Autodesk Inventor part; units mm, degrees
(part 2 of 3)
  spline S117 degree 2 poles (10.1065, 124.379) (9.1972, 124.379) (8.3459, 125.7919) (8.3459, 127.2404) knots 0 0 0 1 2 2 2
  spline S118 degree 2 poles (8.3459, 127.2404) (8.3459, 128.7291) (9.2061, 130.1063) (10.1065, 130.1063) knots 0 0 0 1 2 2 2
  spline S119 degree 2 poles (10.1065, 130.1063) (11.0112, 130.1063) (11.8625, 128.68) (11.8625, 127.2449) knots 0 0 0 1 2 2 2
  spline S120 degree 2 poles (10.9176, 125.569) (11.0246, 125.8409) (11.1138, 126.6788) (11.1138, 127.2449) knots 0 0 0 1 2 2 2
  spline S121 degree 2 poles (11.1138, 127.2449) (11.1138, 127.8109) (11.0246, 128.6444) (10.9132, 128.9252) knots 0 0 0 1 2 2 2
  spline S122 degree 2 poles (10.9132, 128.9252) (10.8018, 129.206) (10.414, 129.4957) (10.1065, 129.4957) knots 0 0 0 1 2 2 2
  spline S123 degree 2 poles (10.1065, 129.4957) (9.7989, 129.4957) (9.4022, 129.206) (9.2864, 128.9163) knots 0 0 0 1 2 2 2
  spline S124 degree 2 poles (9.2864, 128.9163) (9.1749, 128.6355) (9.0947, 127.7797) (9.0947, 127.2404) knots 0 0 0 1 2 2 2
  spline S125 degree 2 poles (9.0947, 127.2404) (9.0947, 126.661) (9.166, 125.8855) (9.2819, 125.5824) knots 0 0 0 1 2 2 2
  spline S126 degree 2 poles (9.2819, 125.5824) (9.3889, 125.2971) (9.7856, 124.9896) (10.1065, 124.9896) knots 0 0 0 1 2 2 2
  spline S127 degree 2 poles (10.1065, 124.9896) (10.4095, 124.9896) (10.8062, 125.2793) (10.9176, 125.569) knots 0 0 0 1 2 2 2
  line L151 (3.304, 115.002) -> (0.6208, 115.002)
  line L152 (0.6208, 115.002) -> (0.6208, 115.5635)
  line L153 (0.6208, 115.5635) -> (1.6192, 115.5635)
  line L154 (1.6192, 115.5635) -> (1.6192, 119.2495)
  line L155 (1.6192, 119.2495) -> (0.6208, 119.2495)
  line L156 (0.6208, 119.2495) -> (0.6208, 119.7532)
  spline S128 degree 2 poles (0.6208, 119.7532) (1.1869, 119.7532) (1.7217, 120.0741) (1.7574, 120.5198) knots 0 0 0 1 2 2 2
  line L157 (1.7574, 120.5198) -> (2.3279, 120.5198)
  line L158 (2.3279, 120.5198) -> (2.3279, 115.5635)
  line L159 (2.3279, 115.5635) -> (3.304, 115.5635)
  line L160 (3.304, 115.5635) -> (3.304, 115.002)
  spline S129 degree 2 poles (7.7387, 117.752) (7.7387, 116.2722) (6.8785, 114.8861) (5.9827, 114.8861) knots 0 0 0 1 2 2 2
  spline S130 degree 2 poles (5.9827, 114.8861) (5.0734, 114.8861) (4.2221, 116.299) (4.2221, 117.7475) knots 0 0 0 1 2 2 2
  spline S131 degree 2 poles (4.2221, 117.7475) (4.2221, 119.2362) (5.0823, 120.6134) (5.9827, 120.6134) knots 0 0 0 1 2 2 2
  spline S132 degree 2 poles (5.9827, 120.6134) (6.8874, 120.6134) (7.7387, 119.1871) (7.7387, 117.752) knots 0 0 0 1 2 2 2
  spline S133 degree 2 poles (6.7938, 116.0761) (6.9008, 116.348) (6.99, 117.1859) (6.99, 117.752) knots 0 0 0 1 2 2 2
  spline S134 degree 2 poles (6.99, 117.752) (6.99, 118.318) (6.9008, 119.1515) (6.7894, 119.4323) knots 0 0 0 1 2 2 2
  spline S135 degree 2 poles (6.7894, 119.4323) (6.678, 119.7131) (6.2902, 120.0028) (5.9827, 120.0028) knots 0 0 0 1 2 2 2
  spline S136 degree 2 poles (5.9827, 120.0028) (5.6751, 120.0028) (5.2784, 119.7131) (5.1626, 119.4233) knots 0 0 0 1 2 2 2
  spline S137 degree 2 poles (5.1626, 119.4233) (5.0511, 119.1426) (4.9709, 118.2868) (4.9709, 117.7475) knots 0 0 0 1 2 2 2
  spline S138 degree 2 poles (4.9709, 117.7475) (4.9709, 117.1681) (5.0422, 116.3926) (5.1581, 116.0895) knots 0 0 0 1 2 2 2
  spline S139 degree 2 poles (5.1581, 116.0895) (5.2651, 115.8042) (5.6617, 115.4967) (5.9827, 115.4967) knots 0 0 0 1 2 2 2
  spline S140 degree 2 poles (5.9827, 115.4967) (6.2857, 115.4967) (6.6824, 115.7864) (6.7938, 116.0761) knots 0 0 0 1 2 2 2
  spline S141 degree 2 poles (11.866, 117.752) (11.866, 116.2722) (11.0058, 114.8861) (10.1099, 114.8861) knots 0 0 0 1 2 2 2
  spline S142 degree 2 poles (10.1099, 114.8861) (9.2006, 114.8861) (8.3494, 116.299) (8.3494, 117.7475) knots 0 0 0 1 2 2 2
  spline S143 degree 2 poles (8.3494, 117.7475) (8.3494, 119.2362) (9.2096, 120.6134) (10.1099, 120.6134) knots 0 0 0 1 2 2 2
  spline S144 degree 2 poles (10.1099, 120.6134) (11.0147, 120.6134) (11.866, 119.1871) (11.866, 117.752) knots 0 0 0 1 2 2 2
  spline S145 degree 2 poles (10.9211, 116.0761) (11.028, 116.348) (11.1172, 117.1859) (11.1172, 117.752) knots 0 0 0 1 2 2 2
  spline S146 degree 2 poles (11.1172, 117.752) (11.1172, 118.318) (11.028, 119.1515) (10.9166, 119.4323) knots 0 0 0 1 2 2 2
  spline S147 degree 2 poles (10.9166, 119.4323) (10.8052, 119.7131) (10.4174, 120.0028) (10.1099, 120.0028) knots 0 0 0 1 2 2 2
  spline S148 degree 2 poles (10.1099, 120.0028) (9.8023, 120.0028) (9.4057, 119.7131) (9.2898, 119.4233) knots 0 0 0 1 2 2 2
  spline S149 degree 2 poles (9.2898, 119.4233) (9.1784, 119.1426) (9.0981, 118.2868) (9.0981, 117.7475) knots 0 0 0 1 2 2 2
  spline S150 degree 2 poles (9.0981, 117.7475) (9.0981, 117.1681) (9.1694, 116.3926) (9.2853, 116.0895) knots 0 0 0 1 2 2 2
  spline S151 degree 2 poles (9.2853, 116.0895) (9.3923, 115.8042) (9.789, 115.4967) (10.1099, 115.4967) knots 0 0 0 1 2 2 2
  spline S152 degree 2 poles (10.1099, 115.4967) (10.413, 115.4967) (10.8096, 115.7864) (10.9211, 116.0761) knots 0 0 0 1 2 2 2
  spline S153 degree 2 poles (0.4266, 108.238) (0.4266, 108.6614) (0.7029, 109.3657) (0.9436, 109.6197) knots 0 0 0 1 2 2 2
  spline S154 degree 2 poles (0.9436, 109.6197) (1.1709, 109.8648) (1.835, 110.1367) (2.1737, 110.1367) knots 0 0 0 1 2 2 2
  spline S155 degree 2 poles (2.1737, 110.1367) (2.5526, 110.1367) (3.1676, 109.8827) (3.395, 109.642) knots 0 0 0 1 2 2 2
  spline S156 degree 2 poles (3.395, 109.642) (3.6802, 109.3389) (3.9922, 108.3584) (3.9922, 107.6051) knots 0 0 0 1 2 2 2
  spline S157 degree 2 poles (3.9922, 107.6051) (3.9922, 106.9232) (3.6847, 105.702) (3.386, 105.2964) knots 0 0 0 1 2 2 2
  spline S158 degree 2 poles (3.386, 105.2964) (3.0696, 104.8685) (2.1782, 104.4183) (1.5275, 104.4183) knots 0 0 0 1 2 2 2
  spline S159 degree 2 poles (1.5275, 104.4183) (1.3804, 104.4183) (1.0461, 104.4495) (0.9035, 104.4941) knots 0 0 0 1 2 2 2
  line L161 (0.9035, 104.4941) -> (0.9035, 105.2028)
  line L162 (0.9035, 105.2028) -> (0.9391, 105.2028)
  spline S160 degree 2 poles (0.9391, 105.2028) (1.0327, 105.1493) (1.4249, 105.0557) (1.6255, 105.0557) knots 0 0 0 1 2 2 2
  spline S161 degree 2 poles (1.6255, 105.0557) (2.3475, 105.0557) (3.1721, 106.0095) (3.23, 106.892) knots 0 0 0 1 2 2 2
  spline S162 degree 2 poles (3.23, 106.892) (2.9359, 106.6914) (2.401, 106.5087) (2.0846, 106.5087) knots 0 0 0 1 2 2 2
  spline S163 degree 2 poles (2.0846, 106.5087) (1.7815, 106.5087) (1.2779, 106.6424) (1.0238, 106.8341) knots 0 0 0 1 2 2 2
  spline S164 degree 2 poles (1.0238, 106.8341) (0.7296, 107.0614) (0.4266, 107.7522) (0.4266, 108.238) knots 0 0 0 1 2 2 2
  spline S165 degree 2 poles (3.2479, 107.77) (3.2479, 108.3272) (3.0428, 109.0314) (2.8601, 109.223) knots 0 0 0 1 2 2 2
  spline S166 degree 2 poles (2.8601, 109.223) (2.6997, 109.4013) (2.3654, 109.535) (2.1693, 109.535) knots 0 0 0 1 2 2 2
  spline S167 degree 2 poles (2.1693, 109.535) (1.7146, 109.535) (1.1753, 108.8843) (1.1753, 108.2692) knots 0 0 0 1 2 2 2
  spline S168 degree 2 poles (1.1753, 108.2692) (1.1753, 107.9216) (1.3536, 107.4714) (1.5497, 107.311) knots 0 0 0 1 2 2 2
  spline S169 degree 2 poles (1.5497, 107.311) (1.6924, 107.1951) (2.0445, 107.1193) (2.2495, 107.1193) knots 0 0 0 1 2 2 2
  spline S170 degree 2 poles (2.2495, 107.1193) (2.4857, 107.1193) (3.0295, 107.2842) (3.2345, 107.4224) knots 0 0 0 1 2 2 2
  spline S171 degree 2 poles (3.2345, 107.4224) (3.239, 107.4759) (3.2479, 107.6586) (3.2479, 107.77) knots 0 0 0 1 2 2 2
  spline S172 degree 2 poles (8.1283, 107.2753) (8.1283, 105.7956) (7.2681, 104.4094) (6.3723, 104.4094) knots 0 0 0 1 2 2 2
  spline S173 degree 2 poles (6.3723, 104.4094) (5.463, 104.4094) (4.6117, 105.8223) (4.6117, 107.2708) knots 0 0 0 1 2 2 2
  spline S174 degree 2 poles (4.6117, 107.2708) (4.6117, 108.7595) (5.4719, 110.1367) (6.3723, 110.1367) knots 0 0 0 1 2 2 2
  spline S175 degree 2 poles (6.3723, 110.1367) (7.277, 110.1367) (8.1283, 108.7105) (8.1283, 107.2753) knots 0 0 0 1 2 2 2
  spline S176 degree 2 poles (7.1834, 105.5994) (7.2904, 105.8713) (7.3796, 106.7093) (7.3796, 107.2753) knots 0 0 0 1 2 2 2
  spline S177 degree 2 poles (7.3796, 107.2753) (7.3796, 107.8413) (7.2904, 108.6748) (7.179, 108.9556) knots 0 0 0 1 2 2 2
  spline S178 degree 2 poles (7.179, 108.9556) (7.0676, 109.2364) (6.6798, 109.5261) (6.3723, 109.5261) knots 0 0 0 1 2 2 2
  spline S179 degree 2 poles (6.3723, 109.5261) (6.0647, 109.5261) (5.6681, 109.2364) (5.5522, 108.9467) knots 0 0 0 1 2 2 2
  spline S180 degree 2 poles (5.5522, 108.9467) (5.4407, 108.6659) (5.3605, 107.8101) (5.3605, 107.2708) knots 0 0 0 1 2 2 2
  spline S181 degree 2 poles (5.3605, 107.2708) (5.3605, 106.6914) (5.4318, 105.9159) (5.5477, 105.6128) knots 0 0 0 1 2 2 2
  spline S182 degree 2 poles (5.5477, 105.6128) (5.6547, 105.3276) (6.0514, 105.02) (6.3723, 105.02) knots 0 0 0 1 2 2 2
  spline S183 degree 2 poles (6.3723, 105.02) (6.6753, 105.02) (7.072, 105.3097) (7.1834, 105.5994) knots 0 0 0 1 2 2 2
  spline S184 degree 2 poles (2.2406, 94.3871) (1.8305, 94.3871) (1.1575, 94.6323) (0.9213, 94.8596) knots 0 0 0 1 2 2 2
  spline S185 degree 2 poles (0.9213, 94.8596) (0.6895, 95.0824) (0.4488, 95.6886) (0.4488, 96.0318) knots 0 0 0 1 2 2 2
  spline S186 degree 2 poles (0.4488, 96.0318) (0.4488, 96.4775) (0.9257, 97.2263) (1.3804, 97.4491) knots 0 0 0 1 2 2 2
  line L163 (1.3804, 97.4491) -> (1.3804, 97.4714)
  spline S187 degree 2 poles (1.3804, 97.4714) (0.9748, 97.7076) (0.5826, 98.2692) (0.5826, 98.6882) knots 0 0 0 1 2 2 2
  spline S188 degree 2 poles (0.5826, 98.6882) (0.5826, 99.3077) (1.5185, 100.1367) (2.2406, 100.1367) knots 0 0 0 1 2 2 2
  spline S189 degree 2 poles (2.2406, 100.1367) (2.9894, 100.1367) (3.8941, 99.3523) (3.8941, 98.7372) knots 0 0 0 1 2 2 2
  spline S190 degree 2 poles (3.8941, 98.7372) (3.8941, 98.3673) (3.4618, 97.6452) (3.0562, 97.4402) knots 0 0 0 1 2 2 2
  line L164 (3.0562, 97.4402) -> (3.0562, 97.4179)
  spline S191 degree 2 poles (3.0562, 97.4179) (3.5376, 97.1951) (4.0323, 96.5533) (4.0323, 96.0452) knots 0 0 0 1 2 2 2
  spline S192 degree 2 poles (4.0323, 96.0452) (4.0323, 95.3409) (3.0072, 94.3871) (2.2406, 94.3871) knots 0 0 0 1 2 2 2
  spline S193 degree 2 poles (3.2746, 95.9738) (3.2746, 96.3126) (3.0072, 96.7137) (2.6283, 96.9187) knots 0 0 0 1 2 2 2
  spline S194 degree 2 poles (2.6283, 96.9187) (2.5035, 96.99) (2.0846, 97.155) (1.8216, 97.2619) knots 0 0 0 1 2 2 2
  spline S195 degree 2 poles (1.8216, 97.2619) (1.5185, 97.0614) (1.1932, 96.4641) (1.1932, 96.0853) knots 0 0 0 1 2 2 2
  spline S196 degree 2 poles (1.1932, 96.0853) (1.1932, 95.5861) (1.7949, 94.9353) (2.2495, 94.9353) knots 0 0 0 1 2 2 2
  spline S197 degree 2 poles (2.2495, 94.9353) (2.713, 94.9353) (3.2746, 95.4925) (3.2746, 95.9738) knots 0 0 0 1 2 2 2
  spline S198 degree 2 poles (3.1721, 98.7283) (3.1721, 99.0982) (2.6774, 99.593) (2.2361, 99.593) knots 0 0 0 1 2 2 2
  spline S199 degree 2 poles (2.2361, 99.593) (1.835, 99.593) (1.3224, 99.1517) (1.3224, 98.7729) knots 0 0 0 1 2 2 2
  spline S200 degree 2 poles (1.3224, 98.7729) (1.3224, 98.501) (1.5854, 98.1221) (1.8484, 97.9706) knots 0 0 0 1 2 2 2
  spline S201 degree 2 poles (1.8484, 97.9706) (1.9598, 97.9082) (2.4322, 97.6898) (2.6239, 97.6274) knots 0 0 0 1 2 2 2
  spline S202 degree 2 poles (2.6239, 97.6274) (2.9448, 97.8725) (3.1721, 98.394) (3.1721, 98.7283) knots 0 0 0 1 2 2 2
  spline S203 degree 2 poles (8.1283, 97.2619) (8.1283, 95.7822) (7.2681, 94.396) (6.3723, 94.396) knots 0 0 0 1 2 2 2
  spline S204 degree 2 poles (6.3723, 94.396) (5.463, 94.396) (4.6117, 95.8089) (4.6117, 97.2575) knots 0 0 0 1 2 2 2
  spline S205 degree 2 poles (4.6117, 97.2575) (4.6117, 98.7461) (5.4719, 100.1234) (6.3723, 100.1234) knots 0 0 0 1 2 2 2
  spline S206 degree 2 poles (6.3723, 100.1234) (7.277, 100.1234) (8.1283, 98.6971) (8.1283, 97.2619) knots 0 0 0 1 2 2 2
  spline S207 degree 2 poles (7.1834, 95.5861) (7.2904, 95.858) (7.3796, 96.6959) (7.3796, 97.2619) knots 0 0 0 1 2 2 2
  spline S208 degree 2 poles (7.3796, 97.2619) (7.3796, 97.828) (7.2904, 98.6614) (7.179, 98.9422) knots 0 0 0 1 2 2 2
  spline S209 degree 2 poles (7.179, 98.9422) (7.0676, 99.223) (6.6798, 99.5127) (6.3723, 99.5127) knots 0 0 0 1 2 2 2
  spline S210 degree 2 poles (6.3723, 99.5127) (6.0647, 99.5127) (5.6681, 99.223) (5.5522, 98.9333) knots 0 0 0 1 2 2 2
  spline S211 degree 2 poles (5.5522, 98.9333) (5.4407, 98.6525) (5.3605, 97.7968) (5.3605, 97.2575) knots 0 0 0 1 2 2 2
  spline S212 degree 2 poles (5.3605, 97.2575) (5.3605, 96.6781) (5.4318, 95.9025) (5.5477, 95.5994) knots 0 0 0 1 2 2 2
  spline S213 degree 2 poles (5.5477, 95.5994) (5.6547, 95.3142) (6.0514, 95.0067) (6.3723, 95.0067) knots 0 0 0 1 2 2 2
  spline S214 degree 2 poles (6.3723, 95.0067) (6.6753, 95.0067) (7.072, 95.2964) (7.1834, 95.5861) knots 0 0 0 1 2 2 2
  line L165 (4.0323, 89.2007) -> (1.6522, 84.5253)
  line L166 (1.6522, 84.5253) -> (0.8678, 84.5253)
  line L167 (0.8678, 84.5253) -> (3.3816, 89.379)
  line L168 (3.3816, 89.379) -> (0.5424, 89.379)
  line L169 (0.5424, 89.379) -> (0.5424, 90.0253)
  line L170 (0.5424, 90.0253) -> (4.0323, 90.0253)
  line L171 (4.0323, 90.0253) -> (4.0323, 89.2007)
  spline S215 degree 2 poles (8.1283, 87.2753) (8.1283, 85.7956) (7.2681, 84.4094) (6.3723, 84.4094) knots 0 0 0 1 2 2 2
  spline S216 degree 2 poles (6.3723, 84.4094) (5.463, 84.4094) (4.6117, 85.8223) (4.6117, 87.2708) knots 0 0 0 1 2 2 2
  spline S217 degree 2 poles (4.6117, 87.2708) (4.6117, 88.7595) (5.4719, 90.1367) (6.3723, 90.1367) knots 0 0 0 1 2 2 2
  spline S218 degree 2 poles (6.3723, 90.1367) (7.277, 90.1367) (8.1283, 88.7105) (8.1283, 87.2753) knots 0 0 0 1 2 2 2
  spline S219 degree 2 poles (7.1834, 85.5994) (7.2904, 85.8713) (7.3796, 86.7093) (7.3796, 87.2753) knots 0 0 0 1 2 2 2
  spline S220 degree 2 poles (7.3796, 87.2753) (7.3796, 87.8413) (7.2904, 88.6748) (7.179, 88.9556) knots 0 0 0 1 2 2 2
  spline S221 degree 2 poles (7.179, 88.9556) (7.0676, 89.2364) (6.6798, 89.5261) (6.3723, 89.5261) knots 0 0 0 1 2 2 2
  spline S222 degree 2 poles (6.3723, 89.5261) (6.0647, 89.5261) (5.6681, 89.2364) (5.5522, 88.9467) knots 0 0 0 1 2 2 2
  spline S223 degree 2 poles (5.5522, 88.9467) (5.4407, 88.6659) (5.3605, 87.8101) (5.3605, 87.2708) knots 0 0 0 1 2 2 2
  spline S224 degree 2 poles (5.3605, 87.2708) (5.3605, 86.6914) (5.4318, 85.9159) (5.5477, 85.6128) knots 0 0 0 1 2 2 2
  spline S225 degree 2 poles (5.5477, 85.6128) (5.6547, 85.3276) (6.0514, 85.02) (6.3723, 85.02) knots 0 0 0 1 2 2 2
  spline S226 degree 2 poles (6.3723, 85.02) (6.6753, 85.02) (7.072, 85.3097) (7.1834, 85.5994) knots 0 0 0 1 2 2 2
  spline S227 degree 2 poles (4.0546, 76.3081) (4.0546, 75.8847) (3.7738, 75.1671) (3.5376, 74.9264) knots 0 0 0 1 2 2 2
  spline S228 degree 2 poles (3.5376, 74.9264) (3.2924, 74.6724) (2.6774, 74.4094) (2.3074, 74.4094) knots 0 0 0 1 2 2 2
  spline S229 degree 2 poles (2.3074, 74.4094) (1.9375, 74.4094) (1.3269, 74.659) (1.0951, 74.9086) knots 0 0 0 1 2 2 2
  spline S230 degree 2 poles (1.0951, 74.9086) (0.8099, 75.2072) (0.489, 76.2101) (0.489, 76.941) knots 0 0 0 1 2 2 2
  spline S231 degree 2 poles (0.489, 76.941) (0.489, 77.6586) (0.7831, 78.813) (1.0907, 79.2409) knots 0 0 0 1 2 2 2
  spline S232 degree 2 poles (1.0907, 79.2409) (1.3893, 79.6598) (2.3342, 80.1278) (2.9537, 80.1278) knots 0 0 0 1 2 2 2
  spline S233 degree 2 poles (2.9537, 80.1278) (3.1364, 80.1278) (3.4574, 80.0922) (3.5777, 80.052) knots 0 0 0 1 2 2 2
  line L172 (3.5777, 80.052) -> (3.5777, 79.3434)
  line L173 (3.5777, 79.3434) -> (3.5465, 79.3434)
  spline S234 degree 2 poles (3.5465, 79.3434) (3.444, 79.3969) (3.0696, 79.4905) (2.8557, 79.4905) knots 0 0 0 1 2 2 2
  spline S235 degree 2 poles (2.8557, 79.4905) (2.1693, 79.4905) (1.3269, 78.5634) (1.2467, 77.6541) knots 0 0 0 1 2 2 2
  spline S236 degree 2 poles (1.2467, 77.6541) (1.5096, 77.8369) (2.0623, 78.0375) (2.3921, 78.0375) knots 0 0 0 1 2 2 2
  spline S237 degree 2 poles (2.3921, 78.0375) (2.713, 78.0375) (3.1944, 77.9082) (3.4574, 77.7121) knots 0 0 0 1 2 2 2
  spline S238 degree 2 poles (3.4574, 77.7121) (3.7604, 77.4848) (4.0546, 76.7806) (4.0546, 76.3081) knots 0 0 0 1 2 2 2
  spline S239 degree 2 poles (3.3058, 76.2769) (3.3058, 76.6157) (3.1275, 77.0747) (2.9314, 77.2352) knots 0 0 0 1 2 2 2
  spline S240 degree 2 poles (2.9314, 77.2352) (2.7843, 77.3511) (2.4189, 77.4268) (2.2272, 77.4268) knots 0 0 0 1 2 2 2
  spline S241 degree 2 poles (2.2272, 77.4268) (1.9687, 77.4268) (1.4829, 77.2708) (1.2467, 77.1238) knots 0 0 0 1 2 2 2
  spline S242 degree 2 poles (1.2467, 77.1238) (1.2422, 77.0435) (1.2333, 76.892) (1.2333, 76.7761) knots 0 0 0 1 2 2 2
  spline S243 degree 2 poles (1.2333, 76.7761) (1.2333, 76.2056) (1.4561, 75.5058) (1.6255, 75.3231) knots 0 0 0 1 2 2 2
  spline S244 degree 2 poles (1.6255, 75.3231) (1.7815, 75.1493) (2.1202, 75.0111) (2.3119, 75.0111) knots 0 0 0 1 2 2 2
  spline S245 degree 2 poles (2.3119, 75.0111) (2.7576, 75.0111) (3.3058, 75.644) (3.3058, 76.2769) knots 0 0 0 1 2 2 2
  spline S246 degree 2 poles (8.1283, 77.2753) (8.1283, 75.7956) (7.2681, 74.4094) (6.3723, 74.4094) knots 0 0 0 1 2 2 2
  spline S247 degree 2 poles (6.3723, 74.4094) (5.463, 74.4094) (4.6117, 75.8223) (4.6117, 77.2708) knots 0 0 0 1 2 2 2
  spline S248 degree 2 poles (4.6117, 77.2708) (4.6117, 78.7595) (5.4719, 80.1367) (6.3723, 80.1367) knots 0 0 0 1 2 2 2
  spline S249 degree 2 poles (6.3723, 80.1367) (7.277, 80.1367) (8.1283, 78.7105) (8.1283, 77.2753) knots 0 0 0 1 2 2 2
  spline S250 degree 2 poles (7.1834, 75.5994) (7.2904, 75.8713) (7.3796, 76.7093) (7.3796, 77.2753) knots 0 0 0 1 2 2 2
  spline S251 degree 2 poles (7.3796, 77.2753) (7.3796, 77.8413) (7.2904, 78.6748) (7.179, 78.9556) knots 0 0 0 1 2 2 2
  spline S252 degree 2 poles (7.179, 78.9556) (7.0676, 79.2364) (6.6798, 79.5261) (6.3723, 79.5261) knots 0 0 0 1 2 2 2
  spline S253 degree 2 poles (6.3723, 79.5261) (6.0647, 79.5261) (5.6681, 79.2364) (5.5522, 78.9467) knots 0 0 0 1 2 2 2
  spline S254 degree 2 poles (5.5522, 78.9467) (5.4407, 78.6659) (5.3605, 77.8101) (5.3605, 77.2708) knots 0 0 0 1 2 2 2
  spline S255 degree 2 poles (5.3605, 77.2708) (5.3605, 76.6914) (5.4318, 75.9159) (5.5477, 75.6128) knots 0 0 0 1 2 2 2
  spline S256 degree 2 poles (5.5477, 75.6128) (5.6547, 75.3276) (6.0514, 75.02) (6.3723, 75.02) knots 0 0 0 1 2 2 2
  spline S257 degree 2 poles (6.3723, 75.02) (6.6753, 75.02) (7.072, 75.3097) (7.1834, 75.5994) knots 0 0 0 1 2 2 2
  spline S258 degree 2 poles (3.912, 66.2725) (3.912, 65.8758) (3.6579, 65.1983) (3.4262, 64.9487) knots 0 0 0 1 2 2 2
  spline S259 degree 2 poles (3.4262, 64.9487) (3.1944, 64.6991) (2.5035, 64.4094) (2.0757, 64.4094) knots 0 0 0 1 2 2 2
  spline S260 degree 2 poles (2.0757, 64.4094) (1.6834, 64.4094) (0.9168, 64.5832) (0.636, 64.7214) knots 0 0 0 1 2 2 2
  line L174 (0.636, 64.7214) -> (0.636, 65.5014)
  line L175 (0.636, 65.5014) -> (0.6895, 65.5014)
  spline S261 degree 2 poles (0.6895, 65.5014) (0.7742, 65.439) (1.0907, 65.2785) (1.2823, 65.2072) knots 0 0 0 1 2 2 2
  spline S262 degree 2 poles (1.2823, 65.2072) (1.5007, 65.1315) (1.8617, 65.0468) (2.089, 65.0468) knots 0 0 0 1 2 2 2
  spline S263 degree 2 poles (2.089, 65.0468) (2.3119, 65.0468) (2.7309, 65.2072) (2.8824, 65.3811) knots 0 0 0 1 2 2 2
  spline S264 degree 2 poles (2.8824, 65.3811) (3.0206, 65.546) (3.1632, 65.9828) (3.1632, 66.2769) knots 0 0 0 1 2 2 2
  spline S265 degree 2 poles (3.1632, 66.2769) (3.1632, 66.5711) (3.0027, 66.9455) (2.8512, 67.0703) knots 0 0 0 1 2 2 2
  spline S266 degree 2 poles (2.8512, 67.0703) (2.6952, 67.2084) (2.2317, 67.3243) (1.9509, 67.3243) knots 0 0 0 1 2 2 2
  spline S267 degree 2 poles (1.9509, 67.3243) (1.6478, 67.3243) (1.0461, 67.2307) (0.8634, 67.1906) knots 0 0 0 1 2 2 2
  line L176 (0.8634, 67.1906) -> (0.8634, 70.0253)
  line L177 (0.8634, 70.0253) -> (3.8808, 70.0253)
  line L178 (3.8808, 70.0253) -> (3.8808, 69.379)
  line L179 (3.8808, 69.379) -> (1.572, 69.379)
  line L180 (1.572, 69.379) -> (1.572, 67.9127)
  spline S268 degree 2 poles (1.572, 67.9127) (1.7057, 67.9305) (1.9642, 67.9439) (2.0712, 67.9439) knots 0 0 0 1 2 2 2
  spline S269 degree 2 poles (2.0712, 67.9439) (2.4946, 67.9439) (3.0785, 67.8057) (3.3459, 67.6007) knots 0 0 0 1 2 2 2
  spline S270 degree 2 poles (3.3459, 67.6007) (3.6178, 67.3956) (3.912, 66.7717) (3.912, 66.2725) knots 0 0 0 1 2 2 2
  spline S271 degree 2 poles (8.1283, 67.2753) (8.1283, 65.7956) (7.2681, 64.4094) (6.3723, 64.4094) knots 0 0 0 1 2 2 2
  spline S272 degree 2 poles (6.3723, 64.4094) (5.463, 64.4094) (4.6117, 65.8223) (4.6117, 67.2708) knots 0 0 0 1 2 2 2
  spline S273 degree 2 poles (4.6117, 67.2708) (4.6117, 68.7595) (5.4719, 70.1367) (6.3723, 70.1367) knots 0 0 0 1 2 2 2
  spline S274 degree 2 poles (6.3723, 70.1367) (7.277, 70.1367) (8.1283, 68.7105) (8.1283, 67.2753) knots 0 0 0 1 2 2 2
  spline S275 degree 2 poles (7.1834, 65.5994) (7.2904, 65.8713) (7.3796, 66.7093) (7.3796, 67.2753) knots 0 0 0 1 2 2 2
  spline S276 degree 2 poles (7.3796, 67.2753) (7.3796, 67.8413) (7.2904, 68.6748) (7.179, 68.9556) knots 0 0 0 1 2 2 2
  spline S277 degree 2 poles (7.179, 68.9556) (7.0676, 69.2364) (6.6798, 69.5261) (6.3723, 69.5261) knots 0 0 0 1 2 2 2
  spline S278 degree 2 poles (6.3723, 69.5261) (6.0647, 69.5261) (5.6681, 69.2364) (5.5522, 68.9467) knots 0 0 0 1 2 2 2
  spline S279 degree 2 poles (5.5522, 68.9467) (5.4407, 68.6659) (5.3605, 67.8101) (5.3605, 67.2708) knots 0 0 0 1 2 2 2
  spline S280 degree 2 poles (5.3605, 67.2708) (5.3605, 66.6914) (5.4318, 65.9159) (5.5477, 65.6128) knots 0 0 0 1 2 2 2
  spline S281 degree 2 poles (5.5477, 65.6128) (5.6547, 65.3276) (6.0514, 65.02) (6.3723, 65.02) knots 0 0 0 1 2 2 2
  spline S282 degree 2 poles (6.3723, 65.02) (6.6753, 65.02) (7.072, 65.3097) (7.1834, 65.5994) knots 0 0 0 1 2 2 2
  line L181 (4.0677, 56.76) -> (3.4126, 56.76)
  line L182 (3.4126, 56.76) -> (3.4126, 54.8703)
  line L183 (3.4126, 54.8703) -> (2.7039, 54.8703)
  line L184 (2.7039, 54.8703) -> (2.7039, 56.76)
  line L185 (2.7039, 56.76) -> (0.2748, 56.76)
  line L186 (0.2748, 56.76) -> (0.2748, 57.5356)
  line L187 (0.2748, 57.5356) -> (2.7351, 60.3703)
  line L188 (2.7351, 60.3703) -> (3.4126, 60.3703)
  line L189 (3.4126, 60.3703) -> (3.4126, 57.3528)
  line L190 (3.4126, 57.3528) -> (4.0677, 57.3528)
  line L191 (4.0677, 57.3528) -> (4.0677, 56.76)
  line L192 (2.7039, 57.3528) -> (2.7039, 59.5011)
  line L193 (2.7039, 59.5011) -> (0.8542, 57.3528)
  line L194 (0.8542, 57.3528) -> (2.7039, 57.3528)
  spline S283 degree 2 poles (8.0791, 57.6203) (8.0791, 56.1405) (7.2189, 54.7544) (6.323, 54.7544) knots 0 0 0 1 2 2 2
  spline S284 degree 2 poles (6.323, 54.7544) (5.4138, 54.7544) (4.5625, 56.1673) (4.5625, 57.6158) knots 0 0 0 1 2 2 2
  spline S285 degree 2 poles (4.5625, 57.6158) (4.5625, 59.1045) (5.4227, 60.4817) (6.323, 60.4817) knots 0 0 0 1 2 2 2
  spline S286 degree 2 poles (6.323, 60.4817) (7.2278, 60.4817) (8.0791, 59.0554) (8.0791, 57.6203) knots 0 0 0 1 2 2 2
  spline S287 degree 2 poles (7.1342, 55.9444) (7.2412, 56.2163) (7.3303, 57.0542) (7.3303, 57.6203) knots 0 0 0 1 2 2 2
  spline S288 degree 2 poles (7.3303, 57.6203) (7.3303, 58.1863) (7.2412, 59.0198) (7.1297, 59.3006) knots 0 0 0 1 2 2 2
  spline S289 degree 2 poles (7.1297, 59.3006) (7.0183, 59.5814) (6.6305, 59.8711) (6.323, 59.8711) knots 0 0 0 1 2 2 2
  spline S290 degree 2 poles (6.323, 59.8711) (6.0155, 59.8711) (5.6188, 59.5814) (5.5029, 59.2916) knots 0 0 0 1 2 2 2
  spline S291 degree 2 poles (5.5029, 59.2916) (5.3915, 59.0109) (5.3113, 58.1551) (5.3113, 57.6158) knots 0 0 0 1 2 2 2
  spline S292 degree 2 poles (5.3113, 57.6158) (5.3113, 57.0364) (5.3826, 56.2609) (5.4984, 55.9578) knots 0 0 0 1 2 2 2
  spline S293 degree 2 poles (5.4984, 55.9578) (5.6054, 55.6725) (6.0021, 55.365) (6.323, 55.365) knots 0 0 0 1 2 2 2
  spline S294 degree 2 poles (6.323, 55.365) (6.6261, 55.365) (7.0228, 55.6547) (7.1342, 55.9444) knots 0 0 0 1 2 2 2
  spline S295 degree 2 poles (2.3776, 49.2493) (2.177, 49.2493) (1.7803, 49.1513) (1.5887, 49.0755) knots 0 0 0 1 2 2 2
  spline S296 degree 2 poles (1.5887, 49.0755) (1.4104, 48.9998) (1.1474, 48.8393) (1.0449, 48.768) knots 0 0 0 1 2 2 2
  line L195 (1.0449, 48.768) -> (1.0004, 48.768)
  line L196 (1.0004, 48.768) -> (1.0004, 49.548)
  spline S297 degree 2 poles (1.0004, 49.548) (1.241, 49.6772) (2.0656, 49.8867) (2.4355, 49.8867) knots 0 0 0 1 2 2 2
  spline S298 degree 2 poles (2.4355, 49.8867) (2.8099, 49.8867) (3.3671, 49.7352) (3.5944, 49.5747) knots 0 0 0 1 2 2 2
  spline S299 degree 2 poles (3.5944, 49.5747) (3.835, 49.4009) (4.0846, 48.8972) (4.0846, 48.5585) knots 0 0 0 1 2 2 2
  spline S300 degree 2 poles (4.0846, 48.5585) (4.0846, 48.1039) (3.4874, 47.4175) (3.0684, 47.3284) knots 0 0 0 1 2 2 2
  line L197 (3.0684, 47.3284) -> (3.0684, 47.2749)
  spline S301 degree 2 poles (3.0684, 47.2749) (3.2423, 47.2392) (3.6389, 47.0788) (3.8083, 46.9183) knots 0 0 0 1 2 2 2
  spline S302 degree 2 poles (3.8083, 46.9183) (3.9777, 46.7623) (4.1916, 46.2631) (4.1916, 45.9021) knots 0 0 0 1 2 2 2
  spline S303 degree 2 poles (4.1916, 45.9021) (4.1916, 45.5322) (3.9376, 44.9037) (3.7058, 44.663) knots 0 0 0 1 2 2 2
  spline S304 degree 2 poles (3.7058, 44.663) (3.4651, 44.4135) (2.7832, 44.1549) (2.3509, 44.1549) knots 0 0 0 1 2 2 2
  spline S305 degree 2 poles (2.3509, 44.1549) (1.9363, 44.1549) (1.1252, 44.3555) (0.8488, 44.4937) knots 0 0 0 1 2 2 2
  line L198 (0.8488, 44.4937) -> (0.8488, 45.2737)
  line L199 (0.8488, 45.2737) -> (0.9023, 45.2737)
  spline S306 degree 2 poles (0.9023, 45.2737) (1.1341, 45.1043) (1.9185, 44.7923) (2.3063, 44.7923) knots 0 0 0 1 2 2 2
  spline S307 degree 2 poles (2.3063, 44.7923) (2.5336, 44.7923) (2.9882, 44.9349) (3.1397, 45.0998) knots 0 0 0 1 2 2 2
  spline S308 degree 2 poles (3.1397, 45.0998) (3.2868, 45.2647) (3.4428, 45.657) (3.4428, 45.9556) knots 0 0 0 1 2 2 2
  spline S309 degree 2 poles (3.4428, 45.9556) (3.4428, 46.2542) (3.269, 46.642) (3.113, 46.7534) knots 0 0 0 1 2 2 2
  spline S310 degree 2 poles (3.113, 46.7534) (2.957, 46.8648) (2.5336, 46.9495) (2.284, 46.9495) knots 0 0 0 1 2 2 2
  line L200 (2.284, 46.9495) -> (1.972, 46.9495)
  line L201 (1.972, 46.9495) -> (1.972, 47.5601)
  line L202 (1.972, 47.5601) -> (2.2171, 47.5601)
  spline S311 degree 2 poles (2.2171, 47.5601) (2.7119, 47.5601) (3.3359, 48.0326) (3.3359, 48.4827) knots 0 0 0 1 2 2 2
  spline S312 degree 2 poles (3.3359, 48.4827) (3.3359, 48.6922) (3.1754, 48.9908) (3.0462, 49.08) knots 0 0 0 1 2 2 2
  spline S313 degree 2 poles (3.0462, 49.08) (2.908, 49.1736) (2.5692, 49.2493) (2.3776, 49.2493) knots 0 0 0 1 2 2 2
  spline S314 degree 2 poles (8.4436, 47.0208) (8.4436, 45.5411) (7.5834, 44.1549) (6.6876, 44.1549) knots 0 0 0 1 2 2 2
  spline S315 degree 2 poles (6.6876, 44.1549) (5.7783, 44.1549) (4.927, 45.5678) (4.927, 47.0164) knots 0 0 0 1 2 2 2
  spline S316 degree 2 poles (4.927, 47.0164) (4.927, 48.505) (5.7872, 49.8823) (6.6876, 49.8823) knots 0 0 0 1 2 2 2
  spline S317 degree 2 poles (6.6876, 49.8823) (7.5923, 49.8823) (8.4436, 48.456) (8.4436, 47.0208) knots 0 0 0 1 2 2 2
  spline S318 degree 2 poles (7.4987, 45.345) (7.6057, 45.6169) (7.6949, 46.4548) (7.6949, 47.0208) knots 0 0 0 1 2 2 2
  spline S319 degree 2 poles (7.6949, 47.0208) (7.6949, 47.5869) (7.6057, 48.4203) (7.4943, 48.7011) knots 0 0 0 1 2 2 2
  spline S320 degree 2 poles (7.4943, 48.7011) (7.3829, 48.9819) (6.9951, 49.2716) (6.6876, 49.2716) knots 0 0 0 1 2 2 2
  spline S321 degree 2 poles (6.6876, 49.2716) (6.38, 49.2716) (5.9833, 48.9819) (5.8675, 48.6922) knots 0 0 0 1 2 2 2
  spline S322 degree 2 poles (5.8675, 48.6922) (5.756, 48.4114) (5.6758, 47.5557) (5.6758, 47.0164) knots 0 0 0 1 2 2 2
  spline S323 degree 2 poles (5.6758, 47.0164) (5.6758, 46.437) (5.7471, 45.6614) (5.863, 45.3583) knots 0 0 0 1 2 2 2
  spline S324 degree 2 poles (5.863, 45.3583) (5.97, 45.0731) (6.3667, 44.7656) (6.6876, 44.7656) knots 0 0 0 1 2 2 2
  spline S325 degree 2 poles (6.6876, 44.7656) (6.9906, 44.7656) (7.3873, 45.0553) (7.4987, 45.345) knots 0 0 0 1 2 2 2
  spline S326 degree 2 poles (4.2735, 17.0475) (4.2735, 15.5677) (3.4133, 14.1816) (2.5174, 14.1816) knots 0 0 0 1 2 2 2
  spline S327 degree 2 poles (2.5174, 14.1816) (1.6082, 14.1816) (0.7569, 15.5945) (0.7569, 17.043) knots 0 0 0 1 2 2 2
  spline S328 degree 2 poles (0.7569, 17.043) (0.7569, 18.5317) (1.6171, 19.9089) (2.5174, 19.9089) knots 0 0 0 1 2 2 2
  spline S329 degree 2 poles (2.5174, 19.9089) (3.4222, 19.9089) (4.2735, 18.4826) (4.2735, 17.0475) knots 0 0 0 1 2 2 2
  spline S330 degree 2 poles (3.3286, 15.3716) (3.4356, 15.6435) (3.5247, 16.4814) (3.5247, 17.0475) knots 0 0 0 1 2 2 2
  spline S331 degree 2 poles (3.5247, 17.0475) (3.5247, 17.6135) (3.4356, 18.447) (3.3241, 18.7278) knots 0 0 0 1 2 2 2
  spline S332 degree 2 poles (3.3241, 18.7278) (3.2127, 19.0086) (2.825, 19.2983) (2.5174, 19.2983) knots 0 0 0 1 2 2 2
  spline S333 degree 2 poles (2.5174, 19.2983) (2.2099, 19.2983) (1.8132, 19.0086) (1.6973, 18.7188) knots 0 0 0 1 2 2 2
  spline S334 degree 2 poles (1.6973, 18.7188) (1.5859, 18.4381) (1.5057, 17.5823) (1.5057, 17.043) knots 0 0 0 1 2 2 2
  spline S335 degree 2 poles (1.5057, 17.043) (1.5057, 16.4636) (1.577, 15.6881) (1.6929, 15.385) knots 0 0 0 1 2 2 2
  spline S336 degree 2 poles (1.6929, 15.385) (1.7998, 15.0997) (2.1965, 14.7922) (2.5174, 14.7922) knots 0 0 0 1 2 2 2
  spline S337 degree 2 poles (2.5174, 14.7922) (2.8205, 14.7922) (3.2172, 15.0819) (3.3286, 15.3716) knots 0 0 0 1 2 2 2
  line L203 (4.3195, 33.9241) -> (0.9276, 33.9241)
  line L204 (0.9276, 33.9241) -> (0.9276, 34.7041)
  spline S338 degree 2 poles (0.9276, 34.7041) (1.2931, 35.0472) (1.9438, 35.6846) (2.2558, 36.0278) knots 0 0 0 1 2 2 2
  spline S339 degree 2 poles (2.2558, 36.0278) (2.8843, 36.7186) (3.3434, 37.5477) (3.3434, 37.9889) knots 0 0 0 1 2 2 2
  spline S340 degree 2 poles (3.3434, 37.9889) (3.3434, 38.2207) (3.2007, 38.5683) (3.0715, 38.6797) knots 0 0 0 1 2 2 2
  spline S341 degree 2 poles (3.0715, 38.6797) (2.9422, 38.7912) (2.6035, 38.9026) (2.3985, 38.9026) knots 0 0 0 1 2 2 2
  spline S342 degree 2 poles (2.3985, 38.9026) (2.2024, 38.9026) (1.8012, 38.8045) (1.6185, 38.7288) knots 0 0 0 1 2 2 2
  spline S343 degree 2 poles (1.6185, 38.7288) (1.4625, 38.6664) (1.1728, 38.4881) (1.0836, 38.4257) knots 0 0 0 1 2 2 2
  line L205 (1.0836, 38.4257) -> (1.0435, 38.4257)
  line L206 (1.0435, 38.4257) -> (1.0435, 39.2101)
  spline S344 degree 2 poles (1.0435, 39.2101) (1.2708, 39.3216) (2.0865, 39.54) (2.452, 39.54) knots 0 0 0 1 2 2 2
  spline S345 degree 2 poles (2.452, 39.54) (3.223, 39.54) (4.0921, 38.7243) (4.0921, 38.029) knots 0 0 0 1 2 2 2
  spline S346 degree 2 poles (4.0921, 38.029) (4.0921, 37.7037) (3.9406, 37.1599) (3.8069, 36.9281) knots 0 0 0 1 2 2 2
  spline S347 degree 2 poles (3.8069, 36.9281) (3.6732, 36.6874) (3.2854, 36.215) (3.0715, 35.9877) knots 0 0 0 1 2 2 2
  spline S348 degree 2 poles (3.0715, 35.9877) (2.7238, 35.6088) (1.8725, 34.7977) (1.6185, 34.5614) knots 0 0 0 1 2 2 2
  line L207 (1.6185, 34.5614) -> (4.3195, 34.5614)
  line L208 (4.3195, 34.5614) -> (4.3195, 33.9241)
  spline S349 degree 2 poles (8.4779, 36.6741) (8.4779, 35.1943) (7.6177, 33.8082) (6.7218, 33.8082) knots 0 0 0 1 2 2 2
  spline S350 degree 2 poles (6.7218, 33.8082) (5.8126, 33.8082) (4.9613, 35.2211) (4.9613, 36.6696) knots 0 0 0 1 2 2 2
  spline S351 degree 2 poles (4.9613, 36.6696) (4.9613, 38.1583) (5.8215, 39.5355) (6.7218, 39.5355) knots 0 0 0 1 2 2 2
  spline S352 degree 2 poles (6.7218, 39.5355) (7.6266, 39.5355) (8.4779, 38.1092) (8.4779, 36.6741) knots 0 0 0 1 2 2 2
  spline S353 degree 2 poles (7.533, 34.9982) (7.64, 35.2701) (7.7291, 36.108) (7.7291, 36.6741) knots 0 0 0 1 2 2 2
  spline S354 degree 2 poles (7.7291, 36.6741) (7.7291, 37.2401) (7.64, 38.0736) (7.5285, 38.3544) knots 0 0 0 1 2 2 2
  spline S355 degree 2 poles (7.5285, 38.3544) (7.4171, 38.6352) (7.0293, 38.9249) (6.7218, 38.9249) knots 0 0 0 1 2 2 2
  spline S356 degree 2 poles (6.7218, 38.9249) (6.4143, 38.9249) (6.0176, 38.6352) (5.9017, 38.3455) knots 0 0 0 1 2 2 2
  spline S357 degree 2 poles (5.9017, 38.3455) (5.7903, 38.0647) (5.7101, 37.2089) (5.7101, 36.6696) knots 0 0 0 1 2 2 2
  spline S358 degree 2 poles (5.7101, 36.6696) (5.7101, 36.0902) (5.7814, 35.3147) (5.8973, 35.0116) knots 0 0 0 1 2 2 2
  spline S359 degree 2 poles (5.8973, 35.0116) (6.0042, 34.7263) (6.4009, 34.4188) (6.7218, 34.4188) knots 0 0 0 1 2 2 2
  spline S360 degree 2 poles (6.7218, 34.4188) (7.0249, 34.4188) (7.4216, 34.7085) (7.533, 34.9982) knots 0 0 0 1 2 2 2
  point P0 (190.5653, 91.5)
  point P1 (8.4853, 17.25)
  dimension "d94" = 1
  constraints: 14 end point, 3 midpoint, 2 parallel, 2 perpendicular, 2 point on line, 1 horizontal, 30 other
  measures "d94" distance of L61.end L62.end
extrude "Extrusion14" add sketch "Skizze14" along normal blind 1 contours L61 L62 L63 L67 | L68 L69 L70 L71 L72 L73 S0 L74 L75 L76 L77 | S1 S2 S3 S4 S5 S6 S7 L78 L79 S8 S9 S10 S11 S12 | S20 S21 S22 S23 | L80 L81 L82 L83 L84 L85 S32 L86 L87 L88 L89 | S33 S34 S35 L90 L91 S36 S37 S38 S39 S40 S41 S42 L92 L93 L94 L95 L96 S43 S44 S45 | S46 S47 S48 S49 | L97 L98 L99 L100 L101 L102 S58 L103 L104 L105 L106 | S59 S60 L107 L108 S61 S62 S63 S64 L109 S65 S66 S67 S68 S69 L110 L111 S70 S71 S72 S73 S74 L112 L113 L114 S75 S76 S77 | S78 S79 S80 S81 | L115 L116 L117 L118 L119 L120 S90 L121 L122 L123 L124 | L125 L126 S91 S92 S93 S94 S95 S96 L127 L128 S97 S98 S99 S100 S101 L129 L130 | S102 S103 S104 S105 | L131 L132 L133 L134 L135 L136 S114 L137 L138 L139 L140 | L141 L142 L143 L144 L145 L146 S115 L147 L148 L149 L150 | S116 S117 S118 S119 | L151 L152 L153 L154 L155 L156 S128 L157 L158 L159 L160 | S129 S130 S131 S132 | S141 S142 S143 S144 | S153 S154 S155 S156 S157 S158 S159 L161 L162 S160 S161 S162 S163 S164 | S172 S173 S174 S175 | S184 S185 S186 L163 S187 S188 S189 S190 L164 S191 S192 | S203 S204 S205 S206 | L165 L166 L167 L168 L169 L170 L171 | S215 S216 S217 S218 | S227 S228 S229 S230 S231 S232 S233 L172 L173 S234 S235 S236 S237 S238 | S246 S247 S248 S249 | S258 S259 S260 L174 L175 S261 S262 S263 S264 S265 S266 S267 L176 L177 L178 L179 L180 S268 S269 S270 | S271 S272 S273 S274 | L181 L182 L183 L184 L185 L186 L187 L188 L189 L190 L191 | S283 S284 S285 S286 | S295 S296 L195 L196 S297 S298 S299 S300 L197 S301 S302 S303 S304 S305 L198 L199 S306 S307 S308 S309 S310 L200 L201 L202 S311 S312 S313 | S314 S315 S316 S317 | S326 S327 S328 S329 | L203 L204 S338 S339 S340 S341 S342 S343 L205 L206 S344 S345 S346 S347 S348 L207 L208 | S349 S350 S351 S352
sketch "Skizze17" plane through (-65, -62, 24) normal (0, -1, 0) x (1, 0, 0)
  line L0 (-5, 0) -> (-5, 156.5)
  line L1 (-5, 156.5) -> (-6, 157.5) projected
  line L2 (-5, 156.5) -> (-6, 157.5)
  line L3 (-13.5, 165) -> (-22, 156.5) projected
  line L4 (-6, 157.5) -> (-13.5, 165)
  line L5 (-13.5, 165) -> (-22, 156.5)
  line L6 (-5, 0) -> (-22, 0) projected
  line L7 (-22, 156.5) -> (-22, 0)
  line L8 (-22, 0) -> (-5, 0)
  line L9 (135, 0) -> (135, 156.5)
  line L10 (136, 157.4) -> (135, 156.5) projected
  line L11 (135, 156.5) -> (136, 157.4)
  line L12 (143.9474, 164.5526) -> (136, 157.4) projected
  line L13 (136, 157.4) -> (143.9474, 164.5526)
  line L14 (152, 0) -> (152, 156.5) projected
  line L15 (143.9474, 164.5526) -> (152, 156.5)
  line L16 (136, 0) -> (152, 0) projected
  line L17 (152, 156.5) -> (152, 0)
  line L18 (152, 0) -> (135, 0)
  point P0 (65, -24)
  constraints: 25 end point, 4 collinear, 4 perpendicular, 1 vertical
extrude "Extrusion15" add sketch "Skizze17" against normal blind 3
sketch "Skizze18" plane through (-71, -86.5, 181.5) normal (1, 0, 0) x (0, 0, -1)
  line L0 (-5, 24.5) -> (1, 24.5) projected
  line L1 (0, 24.5) -> (0, 0) projected
  line L2 (0, 24.5) -> (0, 0)
  line L3 (157.5, 0) -> (160.5, 0) projected
  line L4 (0, 0) -> (157.5, 0)
  line L5 (157.5, 24.5) -> (160.5, 24.5) projected
  line L6 (157.5, 0) -> (157.5, 24.5)
  line L7 (-5, 24.5) -> (0, 24.5) projected
  line L8 (157.5, 24.5) -> (0, 24.5)
  point P0 (181.5, 86.5)
  point P1 (1, 24.5)
  constraints: 8 end point, 3 collinear, 1 perpendicular, 1 point on line
extrude "Extrusion16" add sketch "Skizze18" against normal blind 3
sketch "Skizze20" plane through (71, -86.5, 181.4) normal (-1, 0, 0) x (0, 0, 1)
  line L0 (5.1, 24.5) -> (0, 24.5) projected
  line L1 (0, 0) -> (0, 24.5) projected
  line L2 (0, 24.5) -> (0, 0)
  line L3 (-157.4, 0) -> (-157.4, 24.5) projected
  line L4 (0, 0) -> (-157.4, 0)
  line L5 (-157.4, 0) -> (-157.4, 24.5)
  line L6 (-157.4, 24.5) -> (0, 24.5)
  point P0 (-181.4, 86.5)
  constraints: 8 end point, 3 perpendicular, 1 collinear
extrude "Extrusion17" add sketch "Skizze20" against normal blind 3
sketch "Skizze30" plane through (89, -91.5, 0) normal (1, 0, 0) x (0, 0, -1)
  line L0 (0, 0) -> (0, 183) projected
  line L1 (-24, 181) -> (-24, 32.5) projected
  line L2 (0, 183) -> (-24, 183)
  line L3 (-24, 183) -> (-24, 159)
  line L4 (-24, 159) -> (0, 159)
  line L5 (0, 159) -> (0, 183)
  line L6 (-180.5, 183) -> (-180.5, 169.25) projected
  line L7 (-180.5, 183) -> (-156.5, 183)
  line L8 (-156.5, 183) -> (-156.5, 159)
  line L9 (-156.5, 159) -> (-180.5, 159)
  line L10 (-180.5, 159) -> (-180.5, 183)
  line L11 (-24, 0) -> (-180.5, 0) projected
  line L12 (-180.5, 0) -> (-156.5, 0)
  line L13 (-156.5, 0) -> (-156.5, 24)
  line L14 (-156.5, 24) -> (-180.5, 24)
  line L15 (-180.5, 24) -> (-180.5, 0)
  line L16 (0, 0) -> (-24, 0)
  line L17 (-24, 0) -> (-24, 24)
  line L18 (-24, 24) -> (0, 24)
  line L19 (0, 24) -> (0, 0)
  point P0 (0, 91.5)
  point P1 (0, 24)
  dimension "d140" = 24
  dimension "d141" = 24
  dimension "d142" = 24
  dimension "d143" = 24
  dimension "d144" = 24
  dimension "d145" = 24
  dimension "d146" = 24
  constraints: 32 end point, 8 parallel, 4 horizontal, 4 perpendicular, 1 point on line
  measures "d140" distance of L0.end L2.end
  measures "d141" distance of L3.end L2.end
  measures "d142" distance of L6.start L7.end
  measures "d143" distance of L13.end L14.end
  measures "d144" distance of L12.end L13.end
  measures "d145" distance of L17.end L18.end
  measures "d146" distance of L16.end L17.end
extrude "Extrusion20" add sketch "Skizze30" against normal blind 5
sketch "Skizze33" plane through (89, -91.5, 0) normal (1, 0, 0) x (0, 0, -1)
  line L0 (-180.5, 0) -> (-180.5, 183) projected
  line L1 (0, 0) -> (-180.5, 0) projected
  line L2 (0, 183) -> (-180.5, 183) projected
  line L3 (0, 183) -> (-180.5, 183) projected
  line L4 (0, 0) -> (0, 183) projected
  line L5 (-5, 5) -> (-19, 5)
  line L6 (-19, 5) -> (-19, 19)
  line L7 (-19, 19) -> (-5, 19)
  line L8 (-5, 19) -> (-5, 5)
  line L9 (-5, 178) -> (-19, 178)
  line L10 (-19, 178) -> (-19, 164)
  line L11 (-19, 164) -> (-5, 164)
  line L12 (-5, 164) -> (-5, 178)
  line L13 (-175.5, 178) -> (-161.5, 178)
  line L14 (-161.5, 178) -> (-161.5, 164)
  line L15 (-161.5, 164) -> (-175.5, 164)
  line L16 (-175.5, 164) -> (-175.5, 178)
  line L17 (-175.5, 5) -> (-161.5, 5)
  line L18 (-161.5, 5) -> (-161.5, 19)
  line L19 (-161.5, 19) -> (-175.5, 19)
  line L20 (-175.5, 19) -> (-175.5, 5)
  point P0 (0, 91.5)
  point P1 (-32, 183)
  point P2 (-31, 183)
  dimension "d161" = 5
  dimension "d162" = 5
  dimension "d163" = 5
  dimension "d164" = 5
  dimension "d165" = 5
  dimension "d166" = 5
  dimension "d167" = 5
  dimension "d168" = 5
  dimension "d169" = 14
  dimension "d170" = 14
  dimension "d171" = 14
  dimension "d172" = 14
  dimension "d173" = 14
  dimension "d174" = 14
  dimension "d175" = 14
  dimension "d176" = 14
  constraints: 32 end point, 8 parallel, 4 horizontal, 4 perpendicular, 2 point on line
  measures "d161" distance from line of L17.start L0
  measures "d162" distance from line of L1 L17.start
  measures "d163" distance from line of L2 L13.start
  measures "d164" distance from line of L13.start L0
  measures "d165" distance from line of L3 L9.start
  measures "d166" distance from line of L9.start L4
  measures "d167" distance from line of L5.start L1
  measures "d168" distance from line of L5.start L4
  measures "d169" distance of L19.end L17.start
  measures "d170" distance of L18.end L19.end
  measures "d171" distance of L14.end L15.end
  measures "d172" distance of L15.end L13.start
  measures "d173" distance of L9.end L10.end
  measures "d174" distance of L9.start L9.end
  measures "d175" distance of L6.end L7.end
  measures "d176" distance of L5.end L6.end
extrude "Extrusion21" cut sketch "Skizze33" against normal blind 3 contours L5 L6 L7 L8 | L12 L11 L10 L9 | L13 L14 L15 L16 | L20 L19 L18 L17
sketch "Skizze35" plane through (-89, 91.5, 0) normal (0, 1, 0) x (1, 0, 0)
  line L0 (154, -24) -> (24, -24) projected
  line L1 (79, 24) -> (99, 24)
  line L2 (99, 24) -> (99, -24)
  line L3 (99, -24) -> (79, -24)
  line L4 (79, -24) -> (79, 24)
  line L5 (79, 24) -> (99, -24) construction
  line L6 (99, 24) -> (79, -24) construction
  line L7 (78, -24) -> (80, -24)
  line L8 (80, -24) -> (80, 24)
  line L9 (80, 24) -> (78, 24)
  line L10 (78, 24) -> (78, -24)
  line L11 (78, -24) -> (80, 24) construction
  line L12 (80, -24) -> (78, 24) construction
  line L13 (100, -24) -> (98, -24)
  line L14 (98, -24) -> (98, 24)
  line L15 (98, 24) -> (100, 24)
  line L16 (100, 24) -> (100, -24)
  line L17 (13.65, 0) -> (164.35, 0) projected
  line L18 (100, -24) -> (98, 24) construction
  line L19 (98, -24) -> (100, 24) construction
  point P0 (89, 0)
  point P1 (79, 0)
  point P2 (99, 0)
  point P3 (78, 0)
  point P4 (100, 0)
  dimension "d179" = 20
  dimension "d180" = 2
  dimension "d181" = 2
  constraints: 36 end point, 8 midpoint, 6 parallel, 4 point on line, 3 horizontal, 3 perpendicular
  measures "d179" distance of L1.start L1.end
  measures "d180" distance of L14.end L15.end
  measures "d181" distance of L9.end L8.end
extrude "Extrusion22" cut sketch "Skizze35" against normal blind 1 contours L0 L2 L17 L16 | L0 L10 L17 L4
sketch "Skizze36" plane through (-89, 90.5, 0) normal (0, 1, 0) x (1, 0, 0)
  line L0 (78, -24) -> (78, 0) projected
  line L1 (78, 0) -> (79, 0)
  line L2 (79, 0) -> (79, -1)
  line L3 (79, -1) -> (78, -1)
  line L4 (78, -1) -> (78, 0)
  line L5 (13.65, 0) -> (164.35, 0) projected
  line L6 (99, 0) -> (100, 0)
  line L7 (100, 0) -> (100, -1)
  line L8 (100, -1) -> (99, -1)
  line L9 (99, -1) -> (99, 0)
  point P0 (89, 0)
  constraints: 16 end point, 4 parallel, 2 horizontal, 2 perpendicular, 1 point on line
extrude "Extrusion23" cut sketch "Skizze36" against normal blind 20
sketch "Skizze38" plane through (-89, 91.5, 180.5) normal (0, 1, 0) x (1, 0, 0)
  line L0 (24, 156.5) -> (24, 92) projected
  line L1 (154, 156.5) -> (154, 92) projected
  dimension "d186" = 130
  measures "d186" distance between parallel lines of L0 L1
sketch "Skizze40" plane through (77, 91.5, 192.5) normal (0, 0, -1) x (0, -1, 0)
  line L0 (0, 166) -> (0, 154) projected
  line L1 (183, -12) -> (0, -12) projected
  line L2 (0, 166) -> (183, 166)
  line L3 (183, 166) -> (183, -12)
  line L4 (183, -12) -> (0, -12)
  line L5 (0, -12) -> (0, 166)
  point P0 (91.5, 77)
  constraints: 8 end point, 2 parallel, 1 horizontal, 1 perpendicular
extrude "Extrusion25" cut sketch "Skizze40" along normal blind 168.5 and the other way blind 5
sketch "Skizze42" plane through (0, 0, 0) normal (0, 0, -1) x (-1, 0, 0)
  line L0 (-79.15, 73.1454) -> (-79.15, 69.8546)
  line L1 (-82, 74.7909) -> (-79.15, 73.1454)
  line L2 (-79.15, 69.8546) -> (-82, 68.2091)
  line L3 (-82, 68.2091) -> (-84.85, 69.8546)
  line L4 (-84.85, 69.8546) -> (-84.85, 73.1454)
  line L5 (-84.85, 73.1454) -> (-82, 74.7909)
  line L6 (-82, 74.7909) -> (-96.75, 74.7909)
  line L7 (-82, 68.2091) -> (-96.75, 68.2091)
  line L8 (-96.75, 74.7909) -> (-96.75, 68.2091)
  line L9 (-94, 91.5) -> (-70, 91.5) construction
  line L10 (-82, 91.5) -> (-82, -91.5) construction
  line L11 (-70, -91.5) -> (-94, -91.5) construction
  line L12 (-94, -91.5) -> (-94, 91.5) construction
  line L13 (-70, -62) -> (-70, 91.5) construction
  line L14 (-82, 34.7909) -> (-79.15, 33.1454)
  line L15 (-79.15, 33.1454) -> (-79.15, 29.8546)
  line L16 (-79.15, 29.8546) -> (-82, 28.2091)
  line L17 (-82, 28.2091) -> (-84.85, 29.8546)
  line L18 (-84.85, 33.1454) -> (-82, 34.7909)
  line L19 (-84.85, 29.8546) -> (-84.85, 33.1454)
  line L20 (-82, 28.2091) -> (-96.75, 28.2091)
  line L21 (-82, 34.7909) -> (-96.75, 34.7909)
  line L22 (-96.75, 34.7909) -> (-96.75, 28.2091)
  line L23 (-82, -14.7909) -> (-84.85, -13.1454)
  line L24 (-82, -8.2091) -> (-96.75, -8.2091)
  line L25 (-82, -8.2091) -> (-79.15, -9.8546)
  line L26 (-84.85, -9.8546) -> (-82, -8.2091)
  line L27 (-96.75, -8.2091) -> (-96.75, -14.7909)
  line L28 (-82, -14.7909) -> (-96.75, -14.7909)
  line L29 (-84.85, -13.1454) -> (-84.85, -9.8546)
  line L30 (-79.15, -9.8546) -> (-79.15, -13.1454)
  line L31 (-79.15, -13.1454) -> (-82, -14.7909)
  line L32 (-82, -54.7909) -> (-84.85, -53.1454)
  line L33 (-82, -48.2091) -> (-96.75, -48.2091)
  line L34 (-82, -48.2091) -> (-79.15, -49.8546)
  line L35 (-84.85, -49.8546) -> (-82, -48.2091)
  line L36 (-96.75, -48.2091) -> (-96.75, -54.7909)
  line L37 (-82, -54.7909) -> (-96.75, -54.7909)
  line L38 (-84.85, -53.1454) -> (-84.85, -49.8546)
  line L39 (-79.15, -49.8546) -> (-79.15, -53.1454)
  line L40 (-79.15, -53.1454) -> (-82, -54.7909)
  line L41 (0, 91.5) -> (0, -95.2854)
  line L42 (79.15, 73.1454) -> (79.15, 69.8546)
  line L43 (82, 74.7909) -> (79.15, 73.1454)
  line L44 (79.15, 69.8546) -> (82, 68.2091)
  line L45 (82, 68.2091) -> (84.85, 69.8546)
  line L46 (84.85, 69.8546) -> (84.85, 73.1454)
  line L47 (84.85, 73.1454) -> (82, 74.7909)
  line L48 (82, 74.7909) -> (96.75, 74.7909)
  line L49 (96.75, 74.7909) -> (96.75, 68.2091)
  line L50 (94, 91.5) -> (70, 91.5) construction
  line L51 (82, 68.2091) -> (96.75, 68.2091)
  line L52 (82, 34.7909) -> (96.75, 34.7909)
  line L53 (82, 34.7909) -> (79.15, 33.1454)
  line L54 (84.85, 33.1454) -> (82, 34.7909)
  line L55 (96.75, 34.7909) -> (96.75, 28.2091)
  line L56 (82, 28.2091) -> (96.75, 28.2091)
  line L57 (79.15, 33.1454) -> (79.15, 29.8546)
  line L58 (79.15, 29.8546) -> (82, 28.2091)
  line L59 (82, 28.2091) -> (84.85, 29.8546)
  line L60 (70, -62) -> (70, 91.5) construction
  line L61 (82, 91.5) -> (82, -91.5) construction
  line L62 (94, -91.5) -> (94, 91.5) construction
  line L63 (70, -91.5) -> (94, -91.5) construction
  line L64 (84.85, 29.8546) -> (84.85, 33.1454)
  line L65 (82, -8.2091) -> (79.15, -9.8546)
  line L66 (84.85, -9.8546) -> (82, -8.2091)
  line L67 (79.15, -9.8546) -> (79.15, -13.1454)
  line L68 (84.85, -13.1454) -> (84.85, -9.8546)
  line L69 (82, -14.7909) -> (84.85, -13.1454)
  line L70 (79.15, -13.1454) -> (82, -14.7909)
  line L71 (82, -48.2091) -> (79.15, -49.8546)
  line L72 (79.15, -49.8546) -> (79.15, -53.1454)
  line L73 (79.15, -53.1454) -> (82, -54.7909)
  line L74 (82, -8.2091) -> (96.75, -8.2091)
  line L75 (82, -54.7909) -> (84.85, -53.1454)
  line L76 (84.85, -49.8546) -> (82, -48.2091)
  line L77 (84.85, -53.1454) -> (84.85, -49.8546)
  line L78 (96.75, -8.2091) -> (96.75, -14.7909)
  line L79 (82, -14.7909) -> (96.75, -14.7909)
  line L80 (82, -48.2091) -> (96.75, -48.2091)
  line L81 (96.75, -48.2091) -> (96.75, -54.7909)
  line L82 (82, -54.7909) -> (96.75, -54.7909)
  circle A0 centre (82, 71.5) radius 1.7
  circle A1 centre (82, 31.5) radius 1.7
  circle A2 centre (82, -11.5) radius 1.7
  circle A3 centre (82, -51.5) radius 1.7
  circle A4 centre (-82, -51.5) radius 1.7
  circle A5 centre (-82, -11.5) radius 1.7
  circle A6 centre (-82, 31.5) radius 1.7
  circle A7 centre (-82, 71.5) radius 1.7
  point P0 (0, 0)
  point P1 (0, 0)
  point P2 (-82, 71.5)
  point P3 (-82, 71.5)
  point P4 (-82, -51.5)
  point P5 (-82, 31.5)
  point P6 (-82, -11.5)
  point P7 (-82, 31.5)
  point P8 (-82, -11.5)
  point P9 (-82, -11.5)
  point P10 (-82, -11.5)
  point P11 (82, 71.5)
  point P12 (82, 31.5)
  point P13 (82, -11.5)
  point P14 (82, -51.5)
  point P15 (82, -51.5)
  point P16 (82, -51.5)
  point P17 (82, -11.5)
  point P18 (82, -11.5)
  point P19 (82, -11.5)
  point P20 (82, -51.5)
  point P21 (82, 31.5)
  point P22 (82, -11.5)
  point P23 (82, -51.5)
  point P24 (-82, -51.5)
  point P25 (-82, -11.5)
  point P26 (-82, 31.5)
  point P27 (-82, 71.5)
  point P28 (-82, 71.5)
  point P29 (-82, 71.5)
  dimension "d202" = 5.7
  dimension "d203" = 12
  dimension "d204" = 12
  dimension "d205" = 20
  dimension "d206" = 40
  dimension "d207" = 40
  dimension "d208" = 40
  dimension "d209" = 5.7
  dimension "d210" = 5.7
  dimension "d211" = 5.7
  dimension "d212" = 3.4
  dimension "d213" = 3.4
  dimension "d214" = 3.4
  dimension "d215" = 3.4
  dimension "d216" = 3.4
  dimension "d217" = 3.4
  dimension "d218" = 3.4
  dimension "d219" = 3.4
  dimension "d220" = 0
  dimension "d221" = 0
  constraints: 166 end point, 8 centre point, 8 point on line, 3 midpoint, 2 coincident, 1 parallel, 1 vertical, 52 other
  measures "d202" distance between parallel lines of L0 L4
  measures "d203" distance between parallel lines of L12 L10
  measures "d204" distance between parallel lines of L10 L13
  measures "d205" distance from line of L9 point (-82, 71.5)
  measures "d206" distance of L10.end point (-82, -51.5)
  measures "d207" distance of point (-82, 31.5) point (-82, 71.5)
  measures "d208" distance of point (-82, -51.5) point (-82, -11.5)
  measures "d209" distance between parallel lines of L15 L19
  measures "d210" distance between parallel lines of L30 L29
  measures "d211" distance between parallel lines of L39 L38
  measures "d212" diameter of A0
  measures "d213" diameter of A1
  measures "d214" diameter of A2
  measures "d215" diameter of A3
  measures "d216" diameter of A4
  measures "d217" diameter of A5
  measures "d218" diameter of A6
  measures "d219" diameter of A7
  measures "d220" distance of point (-82, 71.5) point (-82, 71.5)
  measures "d221" distance of point (82, 71.5) point (82, 71.5)
extrude "Extrusion26" cut sketch "Skizze42" against normal through all contours A0 | A1 | A2 | A3 | A4 | A5 | A6 | A7